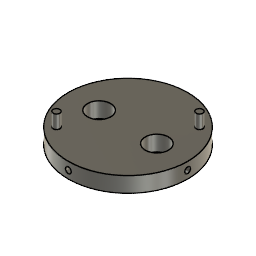
valvedoor v0.2 (Autodesk Fusion 360 design; units mm, degrees)
Autodesk Fusion 360 part; units mm, degrees
sketch "Sketch1" plane through (0, 0, 0) normal (0, 0, 1) x (1, 0, 0)
  circle A0 centre (0, 0) radius 31
  circle A1 centre (-18.5616, -18.5616) radius 1.75
  circle A2 centre (18.5616, 18.5616) radius 1.75
  circle A3 centre (-15, 0) radius 5
  line L0 (-18.5616, -18.5616) -> (-18.5616, -16.8116)
  circle A4 centre (15, 0) radius 5
  line L1 (0, 0) -> (0, 31)
  line L2 (0, 0) -> (31, 0)
  dimension "d1" = 62
  dimension "d6" = 3.5
  dimension "d10" = 15
  dimension "d11" = 10
  constraint coincident A0.centre L1.start
  constraint vertical L0
  constraint coincident A1.centre L0.start
  constraint coincident A1 L0.end
  constraint coincident A0 L1.end
  constraint vertical L1
  constraint coincident A0 L2.end
  constraint perpendicular L1 L2
  measures "d1" diameter of A0
  measures "d6" diameter of A1
  measures "d10" distance of A0.centre A3.centre
  measures "d11" diameter of A3
extrude "Extrude1" add sketch "Sketch1" along normal blind 8 contours A0 A4 L1 L2 | A0 A4 L1 L2
ref_plane "WorkPlane1" through (0, 31, 0) normal (0, 1, 0) x (0, 0, 1)
sketch "Sketch2" plane through (0, 31, 0) normal (0, 1, 0) x (1, 0, 0)
  line L0 (0, 0) -> (0, -2.4162)
  circle A0 centre (0, -4.0162) radius 1.5
  dimension "d27" = 3
  constraint coincident L0.start origin
  constraint vertical L0
  measures "d27" diameter of A0
hole "Hole2" at (-15, 0, 8) direction (0, 0, -1) diameter 12 depth 18 tip angle 180
hole "Hole3" at (15, 0, 8) direction (0, 0, -1) diameter 12 depth 18 tip angle 180
hole "Hole4" at (0, 31, 4.0162) direction (0, -1, 0) diameter 3 depth 6 tip angle 180
pattern_circular "C-Pattern2" count 4 over 360 about axis through (0, 0, 1.75) along (0, 0, 1) of "Hole4"
extrude "Extrude2" add sketch "Sketch1" along normal blind 15 contours A1 | A2
